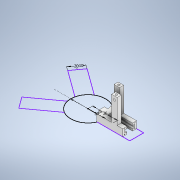
# Autodesk Inventor part: basePart2
Saved by Autodesk Inventor 2021 (Build 250183000, 183)
## iProperties
Created: 2020-11-29
Part Number: basePart2
Material: Generic
Document SubType Name: Modeling
Designer: awitc
Density: 1 g/cm^3
Appearance: Smooth - White
Author: awitc
Autodesk Inventor part; units mm, degrees
ref_plane "YZ Plane" through (0, 0, 0) normal (1, 0, 0) x (0, 1, 0)
ref_plane "XZ Plane" through (0, 0, 0) normal (0, 1, 0) x (-1, 0, 0)
ref_plane "XY Plane" through (0, 0, 0) normal (0, 0, 1) x (1, 0, 0)
sketch "Sketch1" plane through (0, 0, 0) normal (0, 1, 0) x (-1, 0, 0)
  line L0 (0, 0) -> (50, 0) construction
  line L1 (0, 0) -> (50, 0) construction
  line L2 (34.573, 37.4794) -> (12.6591, 21.558)
  line L3 (46.3287, 21.2991) -> (24.4148, 5.3777)
  line L4 (46.3287, -21.2991) -> (24.4148, -5.3777)
  line L5 (34.573, -37.4794) -> (12.6591, -21.558)
  line L6 (-50, -10) -> (-22.9129, -10)
  line L7 (56.6312, -41.145) -> (50.7533, -49.2351)
  line L8 (50.7533, -49.2351) -> (62.509, -33.0548)
  line L9 (62.509, -33.0548) -> (46.3287, -21.2991)
  line L10 (50.7533, -49.2351) -> (34.573, -37.4794)
  line L11 (46.3287, 21.2991) -> (62.509, 33.0548)
  line L12 (62.509, 33.0548) -> (50.7533, 49.2351)
  line L13 (50.7533, 49.2351) -> (34.573, 37.4794)
  line L14 (-50, 10) -> (-70, 10)
  line L15 (-70, 10) -> (-70, -10)
  line L16 (-70, -10) -> (-50, -10)
  line L17 (0, 0) -> (-36, 0)
  circle A0 centre (0, 0) radius 25
  line L18 (-22.9129, 10) -> (-50, 10)
  dimension "d52" = 10
  dimension "d53" = 20
  dimension "d67" = 36
  dimension "d68" = 50
  constraints: 38 end point, 6 point on circle, 5 perpendicular, 4 horizontal, 2 coincident, 1 centre point, 1 parallel, 1 point on line
  measures "d52" distance of L7.start L7.end
  measures "d53" distance of L7.end L8.end
  measures "d67" distance of L17.start L17.end
  measures "d68" diameter of A0
extrude "Extrusion1" add sketch "Sketch1" along normal blind 10
sketch "Sketch8" plane through (-62.509, 0, -33.0548) normal (-0.809, 0, -0.5878) x (-0.5878, 0, 0.809)
  line L0 (-10, 3) -> (-14, 3)
  line L1 (-17, 3) -> (-14, 3)
  line L2 (-3, 3) -> (-3, 7)
  line L3 (-3, 7) -> (-6, 7)
  line L4 (-17, 7) -> (-17, 3)
  line L5 (-10, 0) -> (-6, 0)
  line L6 (14.8816, 0) -> (-15.3777, 0) projected
  line L7 (-6, 0) -> (-6, 3)
  line L8 (-6, 7) -> (-6, 10)
  line L9 (14.8816, 10) -> (-15.3777, 10) projected
  line L10 (-6, 10) -> (-14, 10)
  line L11 (-14, 10) -> (-14, 7)
  line L12 (-14, 3) -> (-14, 0)
  line L13 (-14, 3) -> (-17, 3)
  line L14 (-6, 3) -> (-3, 3)
  line L15 (-14, 7) -> (-17, 7)
  point P0 (-14, 10)
  point P1 (-14, 0)
  dimension "d85" = 3
  dimension "d86" = 7
  dimension "d87" = 14
  dimension "d88" = 4
  dimension "d89" = 4
  dimension "d90" = 8
  constraints: 28 end point, 11 perpendicular, 9 point on line
  measures "d85" distance of L5.start L0.start
  measures "d86" distance of L0.start L1.start
  measures "d87" distance of L1.start L2.start
  measures "d88" distance of L2.start L2.end
  measures "d89" distance of L5.start L5.end
  measures "d90" distance of L8.end L10.end
extrude "Extrusion7" cut sketch "Sketch8" against normal blind 38
sketch "Sketch9" plane through (-50.7533, 0, 49.2351) normal (-0.809, 0, 0.5878) x (0.5878, 0, 0.809)
  line L0 (-10, 3) -> (-14, 3)
  line L1 (-17, 3) -> (-14, 3)
  line L2 (-3, 3) -> (-3, 7)
  line L3 (-3, 7) -> (-6, 7)
  line L4 (-17, 7) -> (-17, 3)
  line L5 (-10, 0) -> (-6, 0)
  line L6 (-6, 0) -> (-6, 3)
  line L7 (-6, 7) -> (-6, 10)
  line L8 (-6, 10) -> (-14, 10)
  line L9 (-14, 10) -> (-14, 7)
  line L10 (-14, 3) -> (-14, 0)
  line L11 (-14, 3) -> (-17, 3)
  line L12 (-6, 3) -> (-3, 3)
  line L13 (-14, 7) -> (-17, 7)
  line L14 (-14, 0) -> (-6, 0)
  line L15 (-6, 3) -> (-3, 3)
  line L16 (-3, 7) -> (-6, 7)
  line L17 (-6, 10) -> (-14, 10)
  line L18 (-4.6223, 10) -> (-34.8816, 10) projected
  line L19 (-14, 10) -> (-14, 7)
  line L20 (-17, 7) -> (-14, 7)
  line L21 (-17, 7) -> (-17, 3)
  line L22 (-14, 3) -> (-17, 3)
  line L23 (-14, 3) -> (-14, 0)
  line L24 (-4.6223, 0) -> (-34.8816, 0) projected
  line L25 (-3, 3) -> (-3, 7)
  line L26 (-6, 7) -> (-6, 10)
  line L27 (-6, 3) -> (-6, 0)
  point P0 (-10, 0)
  point P1 (-15.3777, 0)
  point P2 (-15.3777, 10)
  point P3 (-10, 0)
  dimension "d93" = 3
  dimension "d94" = 7
  dimension "d95" = 14
  dimension "d96" = 4
  dimension "d97" = 4
  dimension "d98" = 8
  constraints: 52 end point, 13 perpendicular, 9 collinear, 7 point on line, 1 parallel
  measures "d93" distance of L5.start L0.start
  measures "d94" distance of L0.start L1.start
  measures "d95" distance of L1.start L2.start
  measures "d96" distance of L2.start L2.end
  measures "d97" distance of L5.start L5.end
  measures "d98" distance of L7.end L8.end
extrude "Extrusion8" cut sketch "Sketch9" against normal blind 38
sketch "Sketch10" plane through (70, 0, 10) normal (1, 0, 0) x (0, 0, -1)
  line L0 (10, 0) -> (10, 3)
  line L1 (10, 3) -> (17, 3)
  line L2 (17, 3) -> (3, 3)
  line L3 (3, 3) -> (6, 3)
  line L4 (6, 3) -> (6, 0)
  line L5 (0, 0) -> (20, 0) projected
  line L6 (6, 0) -> (14, 0)
  line L7 (14, 0) -> (14, 3)
  line L8 (17, 3) -> (17, 7)
  line L9 (17, 7) -> (3, 7)
  line L10 (3, 7) -> (3, 3)
  line L11 (14, 7) -> (14, 10)
  line L12 (0, 10) -> (20, 10) projected
  line L13 (6, 10) -> (14, 10)
  line L14 (6, 10) -> (6, 7)
  dimension "d101" = 3
  dimension "d102" = 7
  dimension "d103" = 14
  dimension "d104" = 3
  dimension "d105" = 8
  dimension "d106" = 4
  constraints: 26 end point, 12 point on line, 6 perpendicular, 1 collinear, 1 parallel, 1 vertical
  measures "d101" distance of L0.start L0.end
  measures "d102" distance of L0.end L1.end
  measures "d103" distance of L1.end L2.end
  measures "d104" distance of L2.end L3.end
  measures "d105" distance of L4.end L6.end
  measures "d106" distance of L1.end L8.end
extrude "Extrusion9" cut sketch "Sketch10" against normal blind 38
sketch "Sketch12" plane through (70, 0, 10) normal (1, 0, 0) x (0, 0, -1)
  line L0 (20, 10) -> (0, 10) projected
  line L1 (43.0548, 0) -> (15.3777, 0) projected
  line L2 (0, 10) -> (20, 10)
  line L3 (20, 10) -> (20, 0)
  line L4 (20, 0) -> (0, 0)
  line L5 (0, 0) -> (0, 10)
  line L6 (0, 10) -> (2.5, 10)
  circle A0 centre (2.5, 8.5) radius 0.5
  circle A1 centre (2.5, 1.5) radius 0.5
  circle A2 centre (17.5, 1.5) radius 0.5
  circle A3 centre (17.5, 8.5) radius 0.5
  point P0 (10, 0)
  point P1 (16.8377, 0)
  point P2 (16.8377, 0)
  dimension "d119" = 20
  dimension "d120" = 2.5
  dimension "d123" = 1
  dimension "d126" = 1
  dimension "d127" = 1
  dimension "d128" = 1
  constraints: 10 end point, 4 centre point, 2 parallel, 2 point on line, 1 horizontal, 1 perpendicular
  measures "d119" distance of L3.end L4.end
  measures "d120" distance of L0.end L6.end
  measures "d123" diameter of A0
  measures "d126" diameter of A1
  measures "d127" diameter of A2
  measures "d128" diameter of A3
extrude "Extrusion14" cut sketch "Sketch12" against normal blind 10
extrude "Extrusion15" cut sketch "Sketch12" against normal blind 14 contours A0 | A1 | A2 | A3
sketch "Sketch13" plane through (-50.7533, 0, -49.2351) normal (-0.809, 0, -0.5878) x (-0.5878, 0, 0.809)
  line L0 (20, 10) -> (0, 10)
  line L1 (0, 10) -> (20, 10)
  line L2 (20, 10) -> (20, 0)
  line L3 (20, 0) -> (0, 0)
  line L4 (0, 0) -> (0, 10)
  line L5 (0, 10) -> (2.5, 10)
  circle A0 centre (2.5, 8.5) radius 0.5
  circle A1 centre (2.5, 1.5) radius 0.5
  circle A2 centre (17.5, 1.5) radius 0.5
  circle A3 centre (17.5, 8.5) radius 0.5
  point P0 (10, 0)
  point P1 (10, 0)
  point P2 (16.8377, 0)
  point P3 (20, 10)
  dimension "d133" = 20
  dimension "d134" = 2.5
  dimension "d135" = 1
  dimension "d136" = 1
  dimension "d137" = 1
  dimension "d138" = 1
  constraints: 12 end point, 4 centre point, 2 parallel, 1 horizontal, 1 perpendicular, 1 point on line
  measures "d133" distance of L2.end L3.end
  measures "d134" distance of L0.end L5.end
  measures "d135" diameter of A0
  measures "d136" diameter of A1
  measures "d137" diameter of A2
  measures "d138" diameter of A3
extrude "Extrusion16" cut sketch "Sketch13" against normal blind 10
extrude "Extrusion17" cut sketch "Sketch13" against normal blind 14 contours A0 | A1 | A2 | A3
sketch "Sketch14" plane through (-62.509, 0, 33.0548) normal (-0.809, 0, 0.5878) x (0.5878, 0, 0.809)
  line L0 (20, 10) -> (0, 10)
  line L1 (0, 10) -> (20, 10)
  line L2 (20, 10) -> (20, 0)
  line L3 (20, 0) -> (0, 0)
  line L4 (0, 0) -> (0, 10)
  line L5 (0, 10) -> (2.5, 10)
  circle A0 centre (2.5, 8.5) radius 0.5
  circle A1 centre (2.5, 1.5) radius 0.5
  circle A2 centre (17.5, 1.5) radius 0.5
  circle A3 centre (17.5, 8.5) radius 0.5
  point P0 (10, 0)
  point P1 (10, 0)
  point P2 (10, 0)
  point P3 (16.8377, 0)
  point P4 (20, 10)
  point P5 (20, 10)
  dimension "d143" = 20
  dimension "d144" = 2.5
  dimension "d145" = 1
  dimension "d146" = 1
  dimension "d147" = 1
  dimension "d148" = 1
  constraints: 12 end point, 4 centre point, 2 parallel, 1 horizontal, 1 perpendicular, 1 point on line
  measures "d143" distance of L2.end L3.end
  measures "d144" distance of L0.end L5.end
  measures "d145" diameter of A0
  measures "d146" diameter of A1
  measures "d147" diameter of A2
  measures "d148" diameter of A3
extrude "Extrusion18" cut sketch "Sketch14" against normal blind 10
extrude "Extrusion19" cut sketch "Sketch14" against normal blind 14 contours A0 | A1 | A2 | A3
sketch "Sketch30" plane through (0, 10, 0) normal (0, 1, 0) x (1, 0, 0)
  line L0 (44, -4) -> (45, -4)
  line L1 (44, -4) -> (52, -4)
  line L2 (52, -4) -> (52, -10)
  line L3 (52, -10) -> (44, -10)
  line L4 (44, -10) -> (44, -4)
  line L5 (33.5, 4) -> (41.5, 4)
  line L6 (41.5, 4) -> (41.5, 10)
  line L7 (41.5, 10) -> (33.5, 10)
  line L8 (33.5, 10) -> (33.5, 4)
  line L9 (-24.7509, -22.9269) -> (-31.2231, -27.6292)
  line L10 (-31.2231, -27.6292) -> (-27.6611, -32.4577)
  line L11 (-27.6611, -32.4577) -> (-21.189, -27.7554)
  line L12 (-21.189, -27.7554) -> (-24.7509, -22.9269)
  line L13 (-50.8922, -32.031) -> (-28.2397, -15.5731) projected
  line L14 (-37.9479, -22.6265) -> (-44.42, -27.3288)
  line L15 (-44.42, -27.3288) -> (-47.9467, -22.4747)
  line L16 (-24.4148, -5.3777) -> (-54.4189, -27.1769) projected
  line L17 (-47.9467, -22.4747) -> (-41.4746, -17.7724)
  line L18 (-41.4746, -17.7724) -> (-37.9479, -22.6265)
  line L19 (-28.2397, 15.5731) -> (-50.8922, 32.031) projected
  line L20 (-50.8922, 32.031) -> (-28.2397, 15.5731) projected
  line L21 (-28.2397, 15.5731) -> (-29.4532, 16.4547)
  line L22 (-29.4532, 16.4547) -> (-32.9799, 11.6006)
  line L23 (-54.4189, 27.1769) -> (-24.4148, 5.3777) projected
  line L24 (-29.4532, 16.4547) -> (-35.9253, 21.157)
  line L25 (-35.9253, 21.157) -> (-39.4521, 16.3029)
  line L26 (-39.4521, 16.3029) -> (-32.9799, 11.6006)
  line L27 (-46.1899, 38.5032) -> (-23.5374, 22.0452) projected
  line L28 (-33.2456, 29.0986) -> (-39.7177, 33.8009)
  line L29 (-39.7177, 33.8009) -> (-36.191, 38.655)
  line L30 (-12.6591, 21.558) -> (-42.6632, 43.3573) projected
  line L31 (-33.2456, 29.0986) -> (-29.7189, 33.9527)
  line L32 (-46.1899, 38.5032) -> (-23.5374, 22.0452) projected
  line L33 (-29.7189, 33.9527) -> (-36.191, 38.655)
  point P0 (0, 0)
  point P1 (32, 4)
  point P2 (42, 10)
  point P3 (34, 10)
  point P4 (41, 10)
  point P5 (-23.5374, -22.0452)
  dimension "d249" = 1
  dimension "d251" = 8
  dimension "d258" = 8
  dimension "d268" = 8
  dimension "d269" = 1.5
  dimension "d270" = 8
  dimension "d271" = 8
  dimension "d278" = 12
  dimension "d279" = 8
  dimension "d282" = 1.5
  dimension "d283" = 8
  dimension "d284" = 12
  dimension "d285" = 8
  constraints: 52 end point, 10 perpendicular, 9 point on line, 4 parallel, 2 horizontal
  measures "d249" distance of L0.start L0.end
  measures "d251" distance of L2.end L3.end
  measures "d258" distance of point (34, 10) point (42, 10)
  measures "d268" distance of L7.end L6.end
  measures "d269" distance of point (-23.537, -22.045) L9.start
  measures "d270" distance of L9.start L9.end
  measures "d271" distance of L10.end L11.end
  measures "d278" distance of L13.end L14.start
  measures "d279" distance of L14.start L14.end
  measures "d282" distance of L19.start L21.end
  measures "d283" distance of L21.end L24.end
  measures "d284" distance of L27.end L28.start
  measures "d285" distance of L28.start L28.end
extrude "Extrusion35" add sketch "Sketch30" along normal blind 35
sketch "Sketch31" plane through (22.9129, 0, -10) normal (0, 0, -1) x (-1, 0, 0)
  line L0 (-9.0871, 45) -> (-19.0871, 45) projected
  circle A0 centre (-14.5871, 28.5) radius 1.5
  point P0 (22.9129, 0)
  dimension "d264" = 3
  constraints: 1 centre point
  measures "d264" diameter of A0
extrude "Extrusion36" cut sketch "Sketch31" against normal up to next
sketch "Sketch32" plane through (32, 7, 4) normal (0, 0, -1) x (-1, 0, 0)
  line L0 (-20, 38) -> (-12, 38) projected
  line L1 (-16, 38) -> (-16, 33)
  circle A0 centre (-16, 33) radius 1.5
  point P0 (32, -7)
  dimension "d253" = 5
  dimension "d254" = 3
  constraints: 2 end point, 1 centre point, 1 coincident, 1 midpoint, 1 vertical
  measures "d253" distance of L1.start L1.end
  measures "d254" diameter of A0
extrude "Extrusion37" cut sketch "Sketch32" against normal up to next
sketch "Sketch33" plane through (-23.5374, 7, 22.0452) normal (-0.5878, 0, -0.809) x (-0.809, 0, 0.5878)
  line L0 (9.4564, 38) -> (1.4564, 38) projected
  line L1 (5.4564, 38) -> (5.4564, 21.5)
  circle A0 centre (5.4564, 21.5) radius 1.5
  point P0 (-32, -7)
  dimension "d286" = 16.5
  dimension "d287" = 3
  constraints: 2 end point, 1 centre point, 1 coincident, 1 midpoint, 1 vertical
  measures "d286" distance of L1.start L1.end
  measures "d287" diameter of A0
sketch "Sketch34" plane through (-24.4148, 0, 5.3777) normal (-0.5878, 0, -0.809) x (-0.809, 0, 0.5878)
  line L0 (29.0871, 45) -> (21.0871, 45) projected
  line L1 (25.0871, 45) -> (25.0871, 40)
  circle A0 centre (25.0871, 40) radius 1.5
  point P0 (-22.9129, 0)
  dimension "d288" = 5
  dimension "d289" = 3
  constraints: 2 end point, 1 centre point, 1 coincident, 1 midpoint, 1 vertical
  measures "d288" distance of L1.start L1.end
  measures "d289" diameter of A0
sketch "Sketch35" plane through (-28.2397, 7, -15.5731) normal (0.5878, 0, -0.809) x (-0.809, 0, -0.5878)
  line L0 (1.5, 38) -> (9.5, 38) projected
  line L1 (5.5, 38) -> (5.5, 21.5)
  circle A0 centre (5.5, 21.5) radius 1.5
  point P0 (-32, -7)
  dimension "d290" = 16.5
  dimension "d291" = 3
  constraints: 2 end point, 1 centre point, 1 coincident, 1 midpoint, 1 vertical
  measures "d290" distance of L1.start L1.end
  measures "d291" diameter of A0
sketch "Sketch36" plane through (-12.6591, 0, -21.558) normal (0.5878, 0, -0.809) x (-0.809, 0, -0.5878)
  line L0 (29.0871, 45) -> (21.0871, 45) projected
  line L1 (25.0871, 45) -> (25.0871, 40)
  circle A0 centre (25.0871, 40) radius 1.5
  point P0 (-22.9129, 0)
  dimension "d292" = 5
  dimension "d293" = 3
  constraints: 2 end point, 1 centre point, 1 coincident, 1 midpoint, 1 vertical
  measures "d292" distance of L1.start L1.end
  measures "d293" diameter of A0
extrude "Extrusion38" cut sketch "Sketch36" against normal up to next
extrude "Extrusion39" cut sketch "Sketch35" against normal up to next
extrude "Extrusion40" cut sketch "Sketch34" against normal up to next
extrude "Extrusion41" cut sketch "Sketch33" against normal up to next
sketch "Sketch37" plane through (0, 10, 0) normal (0, 1, 0) x (1, 0, 0)
  circle A0 centre (0, 0) radius 25
  circle A1 centre (0, 0) radius 22.5
  line L0 (-23.5374, 22.0452) -> (-15.5618, 16.2506)
  line L1 (-23.5374, 22.0452) -> (-13.679, 22.0452) construction
  line L2 (-50.8922, 32.031) -> (-28.2397, 15.5731) projected
  line L3 (-28.2397, 15.5731) -> (-20.2641, 9.7784)
  line L4 (-28.2397, -15.5731) -> (-20.2641, -9.7784)
  line L5 (-23.5374, -22.0452) -> (-15.5618, -16.2506)
  line L6 (60, 4) -> (32, 4) projected
  line L7 (32, 4) -> (22.1416, 4)
  line L8 (32, -4) -> (22.1416, -4)
  circle A2 centre (0, 0) radius 21.25
  line L9 (-20.2641, -9.7784) -> (-19.2354, -9.0311)
  line L10 (-15.5618, -16.2506) -> (-14.5332, -15.5032)
  line L11 (-20.2641, 9.7784) -> (-19.2354, 9.0311)
  line L12 (-15.5618, 16.2506) -> (-14.5332, 15.5032)
  line L13 (22.1416, 4) -> (20.8701, 4)
  line L14 (22.1416, -4) -> (20.8701, -4)
  circle A3 centre (0, 0) radius 22.5
  circle A4 centre (0, 0) radius 21.25
  circle A5 centre (0, 0) radius 20
  line L15 (-19.2354, 9.0311) -> (-18.2046, 8.2821)
  line L16 (-14.5332, 15.5032) -> (-13.5023, 14.7543)
  line L17 (20.8701, -4) -> (19.5959, -4)
  line L18 (20.8701, 4) -> (19.5959, 4)
  line L19 (-14.5332, -15.5032) -> (-13.5023, -14.7543)
  line L20 (-19.2354, -9.0311) -> (-18.2046, -8.2821)
  point P0 (24.6779, -4)
  point P1 (-17.6137, -17.7414)
  point P2 (-22.316, -11.2693)
  point P3 (-22.316, 11.2693)
  point P4 (24.6779, 4)
  point P5 (-17.6137, 17.7414)
  dimension "d302" = 45
  dimension "d303" = 36
  dimension "d306" = 42.5
  dimension "d315" = 45
  dimension "d316" = 42.5
  dimension "d317" = 40
  constraints: 38 end point, 17 point on circle, 7 parallel, 6 centre point, 6 coincident, 3 horizontal, 2 collinear, 1 equal length
  measures "d302" diameter of A1
  measures "d303" angle of L0 L1
  measures "d306" diameter of A2
  measures "d315" diameter of A3
  measures "d316" diameter of A4
  measures "d317" diameter of A5
extrude "Extrusion42" add sketch "Sketch37" along normal blind 23 contours L7 A1 L0 A0 | A0 L5 A1 L8 | L13 A2 L12 A1 | A1 L10 A2 L14 | L3 A1 L4 A0 | L18 A5 L16 A2 | A2 L19 A5 L17 | L11 A2 L9 A1 | L15 A5 L20 A2
sketch "Sketch38" plane through (0, 33, 0) normal (0, 1, 0) x (1, 0, 0)
  line L0 (22.1416, 4) -> (20.8701, 4)
  line L1 (22.1416, -4) -> (20.8701, -4)
  line L2 (24.6779, 4) -> (22.1416, 4)
  line L3 (24.6779, -4) -> (22.1416, -4)
  line L4 (-15.5618, -16.2506) -> (-14.5332, -15.5032)
  line L5 (-15.5618, 16.2506) -> (-14.5332, 15.5032)
  line L6 (-20.2641, -9.7784) -> (-19.2354, -9.0311)
  line L7 (-17.6137, -17.7414) -> (-15.5618, -16.2506)
  line L8 (-22.316, -11.2693) -> (-20.2641, -9.7784)
  line L9 (-20.2641, 9.7784) -> (-19.2354, 9.0311)
  line L10 (-17.6137, 17.7414) -> (-15.5618, 16.2506)
  line L11 (-22.316, 11.2693) -> (-20.2641, 9.7784)
  line L12 (-23.5374, 22.0452) -> (-13.679, 22.0452) construction
  arc A0 (-17.6137, -17.7414) -> (24.6779, -4) centre (0, 0) ccw
  arc A1 (24.6779, 4) -> (-17.6137, 17.7414) centre (0, 0) ccw
  arc A2 (-22.316, 11.2693) -> (-22.316, -11.2693) centre (0, 0) ccw
  line L13 (20.8701, 4) -> (15.8701, 4)
  line L14 (15.8701, 4) -> (15.8701, -4)
  line L15 (15.8701, -4) -> (20.8701, -4)
  line L16 (-14.5332, 15.5032) -> (-10.4881, 12.5643)
  line L17 (-10.4881, 12.5643) -> (-15.1903, 6.0922)
  line L18 (-15.1903, 6.0922) -> (-19.2354, 9.0311)
  line L19 (-19.2354, -9.0311) -> (-15.1903, -6.0922)
  line L20 (-15.1903, -6.0922) -> (-10.4881, -12.5643)
  line L21 (-10.4881, -12.5643) -> (-14.5332, -15.5032)
  circle A3 centre (-22.5, 0) radius 1.5
  circle A4 centre (0, 22.5) radius 1.5
  circle A5 centre (18.2029, 13.2252) radius 1.5
  circle A6 centre (18.2029, -13.2252) radius 1.5
  circle A7 centre (0, -22.5) radius 1.5
  point P0 (-23.5374, -22.0452)
  point P1 (-28.2397, -15.5731)
  dimension "d307" = 36
  dimension "d308" = 5
  dimension "d309" = 5
  dimension "d310" = 3
  dimension "d311" = 3
  dimension "d312" = 3
  dimension "d313" = 3
  dimension "d314" = 3
  constraints: 44 end point, 8 centre point, 6 point on circle, 5 parallel, 4 perpendicular, 3 horizontal, 1 coincident
  measures "d307" angle of L10 L12
  measures "d308" distance of L15.end L14.end
  measures "d309" distance of L16.start L17.start
  measures "d310" diameter of A3
  measures "d311" diameter of A4
  measures "d312" diameter of A5
  measures "d313" diameter of A6
  measures "d314" diameter of A7
extrude "Extrusion43" cut sketch "Sketch38" against normal blind 10 contours A3 | A4 | A5 | A6 | A7
sketch "Sketch39" plane through (0, 45, 0) normal (0, 1, 0) x (1, 0, 0)
  line L0 (-37.9479, -22.6265) -> (-41.4746, -17.7724) projected
  line L1 (-47.9467, -22.4747) -> (-44.42, -27.3288) projected
  line L2 (-31.2231, -27.6292) -> (-27.6611, -32.4577) projected
  circle A0 centre (-42.9473, -22.5506) radius 1.5
  circle A1 centre (-26.2405, -27.6816) radius 1.5
  line L3 (-29.7189, 33.9527) -> (-36.191, 38.655) projected
  line L4 (-39.7177, 33.8009) -> (-33.2456, 29.0986) projected
  line L5 (-29.4532, 16.4547) -> (-35.9253, 21.157) projected
  line L6 (41.5, 10) -> (33.5, 10) projected
  line L7 (33.5, 4) -> (41.5, 4) projected
  line L8 (44, -10) -> (52, -10) projected
  circle A2 centre (48, -7) radius 1.5
  circle A3 centre (37.5, 7) radius 1.5
  circle A4 centre (-34.7183, 33.8768) radius 1.5
  circle A5 centre (-34.4526, 16.3788) radius 1.5
  point P0 (0, 0)
  point P1 (-32.9799, 11.6006)
  point P2 (44, -4)
  dimension "d320" = 3
  dimension "d321" = 3
  dimension "d322" = 3
  dimension "d323" = 3
  dimension "d325" = 3
  constraints: 6 centre point
  measures "d320" diameter of A0
  measures "d321" diameter of A1
  measures "d322" diameter of A2
  measures "d323" diameter of A3
  measures "d325" diameter of A5
extrude "Extrusion44" cut sketch "Sketch39" against normal blind 3
sketch "Sketch40" plane through (0, 33, 0) normal (0, 1, 0) x (1, 0, 0)
  circle A0 centre (0, 0) radius 25
  circle A1 centre (0, 0) radius 91.0936
  line L0 (33.5, 10) -> (22.9129, 10) projected
  line L1 (22.9129, 10) -> (22.9129, 91.0936)
  line L2 (22.9129, 91.0936) -> (22.9129, 10)
  arc A2 (22.9129, 10) -> (-12.6591, 21.558) centre (0, 0) ccw projected
  line L3 (22.9129, -10) -> (22.9129, -88.1648)
  point P0 (22.9129, 88.1648)
  constraints: 6 end point, 2 coincident, 2 point on line, 1 centre point, 1 perpendicular, 1 point on circle, 3 other
extrude "Extrusion45" cut sketch "Sketch40" along normal through all both and the other way through all contours A0 | A0 L3 A1 L1 picked at (-50.6626, -46.6253)
sketch "Sketch41" plane through (0, 10, 0) normal (0, 1, 0) x (1, 0, 0)
  circle A0 centre (0, 0) radius 25
  arc A1 (22.9129, -10) -> (22.9129, 10) centre (0, 0) ccw projected
  line L0 (25, -3) -> (25, 0)
  line L1 (25, 0) -> (25, 3)
  line L2 (25, 3) -> (25, -3)
  line L3 (20, 4) -> (25, 4)
  line L4 (25, 4) -> (25, -4)
  line L5 (25, -4) -> (20, -4)
  line L6 (19.596, -3) -> (19.596, 4)
  line L7 (19.596, 4) -> (20, 4)
  line L8 (19.596, -3) -> (19.596, -4)
  line L9 (19.596, -4) -> (20, -4)
  point P0 (24.6779, 4)
  point P1 (24.6779, -4)
  dimension "d333" = 3
  dimension "d338" = 8
  constraints: 20 end point, 3 perpendicular, 1 centre point, 1 coincident, 1 horizontal, 1 parallel, 1 point on circle, 1 point on line
  measures "d333" distance of L1.end L1.start
  measures "d338" distance of L3.end L4.end
extrude "Extrusion47" add sketch "Sketch41" against normal blind 10 contours A0 L5 L9 L8 L6 L7 L3 picked at (21.532, 0.3333)
body "Solid1"
